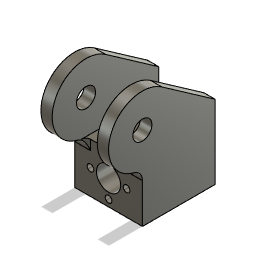
Lead Screw Nut Mount v1 (Autodesk Fusion 360 design; units mm, degrees)
Autodesk Fusion 360 part; units mm, degrees
sketch "Sketch1" plane through (0, 0, 0) normal (0, 0, 1) x (1, 0, 0)
  circle A0 centre (0, 0) radius 5.375
  line L0 (0, 0) -> (0, 45)
  line L1 (0, 0) -> (55, 0)
  line L2 (-15, -11) -> (15, -11)
  line L3 (15, -11) -> (15, 11)
  line L4 (15, 11) -> (-15, 11)
  line L5 (-15, 11) -> (-15, -11)
  circle A1 centre (0, 8) radius 1.5
  circle A2 centre (-8, 0) radius 1.5
  circle A3 centre (0, -8) radius 1.5
  circle A4 centre (8, 0) radius 1.5
  dimension "d5" = 10.75
  dimension "d9" = 3
  dimension "d10" = 8
  dimension "d12" = 360
  dimension "d14" = 3
  dimension "d27" = 30
  constraint coincident A0.centre L0.start
  constraint vertical L0
  constraint perpendicular L0 L1
  constraint horizontal L2
  constraint vertical L3
  constraint horizontal L4
  constraint vertical L5
  constraint symmetric L0 L3 L5
  constraint symmetric L1 L2 L4
  constraint coincident L0 A1.centre
  measures "d5" diameter of A0
  measures "d9" diameter of A1
  measures "d10" distance of A0.centre A1.centre
  measures "d14" distance of L2 A3.centre
  measures "d27" distance of L3 L5
extrude "Extrude1" add sketch "Sketch1" along normal blind 32.25 contours A0 L0 L1 L2 L3 L4 L5 A1 A4 | A0 L0 L1 L3 L4 A1 A4
sketch "Sketch2" plane through (15, 0, 0) normal (1, 0, 0) x (0, 0, -1)
  line L0 (0, -11) -> (0, 11)
  line L1 (0, 11) -> (-32.25, 11)
  line L2 (-32.25, 11) -> (-32.25, -11)
  line L3 (-32.25, -11) -> (0, -11)
  circle A0 centre (-32.25, 26) radius 4.25
  circle A1 centre (-32.25, 26) radius 15
  line L4 (0, 11) -> (0, 21.7299)
  line L5 (0, 21.7299) -> (-23.6464, 38.2873)
  dimension "d20" = 8.5
  dimension "d21" = 15
  dimension "d28" = 30
  dimension "d34" = 125
  constraint concentric A0 A1
  constraint coincident L1.end A1
  constraint coincident L0.end L1.start
  constraint perpendicular L1 L4
  constraint coincident A1 L5.end
  constraint tangent A1 L5
  measures "d20" diameter of A0
  measures "d21" distance of L1 A0.centre
  measures "d28" diameter of A1
  measures "d34" angle of L4 L5
extrude "Extrude2" add sketch "Sketch2" against normal blind 5 contours L1 A1 L4 L5 | A1
ref_plane "WorkPlane1" through (0, 16.75, 24.9478) normal (1, 0, 0) x (0, 1, 0)
mirror "Mirror1" about plane through (0, 16.75, 24.9478) normal (1, 0, 0) of "Extrude2"
fillet "Fillet1" radius 5 2 edges at (-12.5, 11, 32.25) (12.5, 11, 32.25)
fillet "Fillet2" radius 2 1 edges at (-10, 8.8175, 32.25)
equation "Screw_Nut_Dia = 10 mm"
equation "Screw_Nut_bolt_Dia = 3 mm"
equation "Screw_Nut_Bolt_Pattern = 16 mm"
equation "d5 = Screw_Nut_Dia + 0.75 mm"
equation "d9 = Screw_Nut_bolt_Dia"
equation "d10 = Screw_Nut_Bolt_Pattern / 2"
equation "d13 = Screw_Nut_bolt_Dia"
equation "d14 = d13"
equation "d28 = 22 mm + 8 mm"
equation "d34 = 180 deg - 55 deg"
